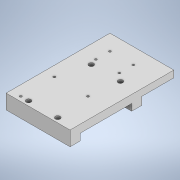
# Autodesk Inventor part: P132SupportCamera
Saved by Autodesk Inventor 2020 (Build 240168000, 168)
## iProperties
Created: 2021-07-29
Part Number: P132SupportCamera
Material: Generic
Document SubType Name: Modeling
Designer: brice.dubuis
Density: 1 g/cm^3
Appearance: Default
Author: brice.dubuis
Autodesk Inventor part; units mm, degrees
ref_plane "YZ Plane" through (0, 0, 0) normal (1, 0, 0) x (0, 1, 0)
ref_plane "XZ Plane" through (0, 0, 0) normal (0, 1, 0) x (-1, 0, 0)
ref_plane "XY Plane" through (0, 0, 0) normal (0, 0, 1) x (1, 0, 0)
sketch "Sketch1" plane through (0, 0, 0) normal (0, 1, 0) x (-1, 0, 0)
  line L0 (0, 0) -> (57, 0)
  line L1 (57, 0) -> (57, -64)
  line L2 (57, -64) -> (0, -64)
  line L3 (0, -64) -> (0, 0)
  dimension "d0" = 57
  dimension "d1" = 64
  constraints: 8 end point, 2 parallel, 1 horizontal, 1 perpendicular
  measures "d0" distance between parallel lines of L3 L1
  measures "d1" distance between parallel lines of L0 L2
extrude "Extrusion1" add sketch "Sketch1" along normal blind 7
sketch "Sketch2" plane through (0, 7, 0) normal (0, 1, 0) x (1, 0, 0)
  line L0 (-57, 64) -> (-57, 0) projected
  line L1 (-57, 0) -> (0, 0) projected
  line L2 (0, 64) -> (-57, 64) projected
  point P0 (-41, 4)
  point P1 (-15, 4)
  point P2 (-41, 60)
  point P3 (-15, 60)
  dimension "d4" = 26
  dimension "d5" = 16
  dimension "d6" = 4
  dimension "d7" = 4
  dimension "d8" = 4
  dimension "d9" = 4
  dimension "d10" = 26
  dimension "d11" = 16
  measures "d4" distance of point (-15, 4) point (-41, 4)
  measures "d5" distance from line of L0 point (-41, 4)
  measures "d6" distance from line of L1 point (-41, 4)
  measures "d7" distance from line of L1 point (-15, 4)
  measures "d8" distance from line of L2 point (-41, 60)
  measures "d9" distance from line of L2 point (-15, 60)
  measures "d10" distance of point (-41, 60) point (-15, 60)
  measures "d11" distance from line of L0 point (-41, 60)
sketch "Sketch3" plane through (0, 0, 0) normal (0, -1, 0) x (1, 0, 0)
  line L0 (0, -64) -> (-57, -64) projected
  line L1 (0, 0) -> (0, -64) projected
  line L2 (-57, -64) -> (0, -64)
  line L3 (0, -64) -> (0, -55)
  line L4 (0, -55) -> (-57, -55)
  line L5 (-57, -55) -> (-57, -64)
  line L6 (-57, -64) -> (-57, 0) projected
  line L7 (-57, 0) -> (0, 0)
  line L8 (0, 0) -> (0, -9)
  line L9 (0, -9) -> (-57, -9)
  line L10 (-57, -9) -> (-57, 0)
  dimension "d12" = 9
  dimension "d13" = 9
  constraints: 16 end point, 4 parallel, 2 horizontal, 2 perpendicular, 2 point on line
  measures "d12" distance between parallel lines of L0 L4
  measures "d13" distance between parallel lines of L7 L9
extrude "Extrusion2" add sketch "Sketch3" along normal blind 6 contours L0 L5 L4 L1 | L9 L6 L7 L1
hole "Hole1" at (-41, 7, -4) at (-15, 7, -4) at (-41, 7, -60) at (-15, 7, -60) direction (0, -1, 0) diameter 4.3 end through all
sketch "Sketch4" plane through (0, 7, 0) normal (0, 1, 0) x (1, 0, 0)
  line L0 (-57, 0) -> (0, 0) projected
  line L1 (-57, 64) -> (-57, 0) projected
  line L2 (0, 0) -> (0, 64) projected
  line L3 (-63.6235, 34) -> (1.4941, 34) construction
  line L4 (-48, -4.864) -> (-48, 68.9429) construction
  point P0 (-48, 4)
  point P1 (-48, 34)
  point P2 (-18, 34)
  dimension "d28" = 4
  dimension "d30" = 9
  dimension "d41" = 30
  dimension "d42" = 30
  constraints: 4 end point, 4 point on line, 1 horizontal, 1 vertical
  measures "d28" distance from line of L0 point (-48, 4)
  measures "d30" distance from line of L1 point (-48, 34)
  measures "d41" distance from line of point (-18, 34) L4
  measures "d42" distance from line of point (-48, 4) L3
hole "Hole2" at (-48, 7, -4) at (-48, 7, -34) at (-18, 7, -34) direction (0, -1, 0) diameter 2.05 end through all
sketch "Sketch5" plane through (0, 7, -64) normal (0, 0, -1) x (-1, 0, 0)
  line L0 (57, -13) -> (57, 0) projected
  line L1 (0, 0) -> (57, 0)
  line L2 (57, 0) -> (57, -6)
  line L3 (57, -6) -> (0, -6)
  line L4 (0, -6) -> (0, 0)
  point P0 (0, -7)
  dimension "d43" = 6
  constraints: 8 end point, 2 parallel, 1 horizontal, 1 perpendicular, 1 point on line
  measures "d43" distance between parallel lines of L3 L1
extrude "Extrusion3" add sketch "Sketch5" along normal blind 28.63
sketch "Sketch6" plane through (0, 7, 0) normal (0, 1, 0) x (1, 0, 0)
  line L0 (-43, 25.0666) -> (-43, 99.5095) construction
  line L1 (-57, 92.63) -> (0, 92.63) projected
  line L2 (-22, 34.9149) -> (-22, 94.8811) construction
  line L3 (-39.656, 66) -> (-5.0422, 66) construction
  line L4 (-57, 0) -> (0, 0) projected
  line L5 (0, 0) -> (0, 92.63) projected
  line L6 (-49.1509, 78.5) -> (-3.6175, 78.5) construction
  point P0 (-43, 66)
  point P1 (-22, 66)
  point P2 (-43, 78.5)
  point P3 (-22, 78.5)
  dimension "d46" = 21
  dimension "d47" = 66
  dimension "d48" = 22
  dimension "d49" = 12.5
  constraints: 8 end point, 8 point on line, 2 perpendicular, 1 horizontal, 1 vertical
  measures "d46" distance between parallel lines of L2 L0
  measures "d47" distance between parallel lines of L4 L3
  measures "d48" distance between parallel lines of L5 L2
  measures "d49" distance between parallel lines of L3 L6
hole "Hole3" at (-43, 7, -66) at (-22, 7, -66) at (-43, 7, -78.5) at (-22, 7, -78.5) direction (0, -1, 0) diameter 1.9 end through all
body "Solid1"
